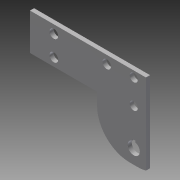
# Autodesk Inventor part: M - arm mount
Saved by Autodesk Inventor 2013 (Build 170138000, 138)
## iProperties
Created: 2013-01-24
Part Number: M - arm mount
Material: Steel
Document SubType Name: Sheet Metal
Designer: Arpan
Density: 7.85 g/cm^3
Sheet Metal Rule: Default
Mass: 87.6442 g
Surface Area: 84.0114 cm^2
Volume: 11.1649 cm^3
Author: Arpan
Autodesk Inventor part; units mm, degrees
ref_plane "YZ Plane" through (0, 0, 0) normal (1, 0, 0) x (0, 1, 0)
ref_plane "XZ Plane" through (0, 0, 0) normal (0, 1, 0) x (-1, 0, 0)
sketch "Sketch1" plane through (0, 0, 0) normal (0, 0, 1) x (1, 0, 0)
  line L0 (-56.9976, 63.5) -> (0, 63.5)
  line L1 (0, 63.5) -> (-7.493, 63.5)
  line L2 (-7.493, 63.5) -> (-7.493, 57.15)
  line L3 (-56.9976, 63.5) -> (-49.5046, 63.5)
  line L4 (-49.5046, 63.5) -> (-49.5046, 57.15)
  line L5 (-56.9976, 63.5) -> (-56.9976, 0)
  line L6 (-56.9976, 0) -> (0, 0)
  line L7 (0, 0) -> (0, 63.5)
  line L8 (-28.4988, 0) -> (-28.4988, 11.1125)
  circle A0 centre (-28.4988, 11.1125) radius 4.7625
  dimension "d3" = 7.493
  dimension "d4" = 6.35
  dimension "d5" = 7.493
  dimension "d19" = 6.35
  dimension "d60" = 63.5
  dimension "d61" = 11.1125
  dimension "d62" = 9.525
  constraints: 18 end point, 3 perpendicular, 2 point on line, 1 centre point, 1 coincident, 1 midpoint, 1 parallel
  measures "d3" distance of L0.end L1.end
  measures "d4" distance of L1.end L2.end
  measures "d5" distance of L0.start L3.end
  measures "d19" distance of L3.end L4.end
  measures "d60" distance of L0.start L5.end
  measures "d61" distance of L8.start L8.end
  measures "d62" diameter of A0
extrude "Plate6" add sketch "Sketch1" along normal blind 3.175
sketch "Sketch6" plane through (0, 0, 0) normal (0, 0, -1) x (-1, 0, 0)
  line L0 (56.9976, 63.5) -> (56.9976, 0) projected
  line L1 (28.4988, 11.1125) -> (27.3076, 11.1125)
  line L2 (28.4988, 11.1125) -> (29.6894, 11.1125)
  circle A0 centre (28.4988, 11.1125) radius 4.7625
  circle A1 centre (28.4988, 11.1125) radius 4.7625 projected
  line L3 (27.3076, 11.1125) -> (29.6888, 11.1125)
  line L4 (29.6888, 11.1125) -> (29.6888, 15.7239)
  line L5 (29.6888, 15.7239) -> (27.3076, 15.7239)
  line L6 (27.3076, 15.7239) -> (27.3076, 11.1125)
  line L7 (27.3076, 15.7239) -> (27.3076, 16.9145)
  line L8 (27.3076, 16.9145) -> (29.6888, 16.9145)
  line L9 (29.6888, 16.9145) -> (29.6888, 15.7239)
  point P0 (27.2012, 15.6948)
  point P1 (30.5454, 15.4129)
  dimension "d82" = 1.1906
  dimension "d86" = 2.3813
  dimension "d87" = 1.1906
  constraints: 18 end point, 6 point on circle, 4 perpendicular, 2 collinear, 2 parallel, 1 centre point, 1 coincident, 1 horizontal
  measures "d82" distance of L1.start L2.end
  measures "d86" distance between parallel lines of L4 L6
  measures "d87" distance of L5.end L7.end
extrude "Cut1" cut sketch "Sketch6" against normal blind 3.175 contours L7 L8 L9 A0 | A0 L5
sketch "Sketch7" plane through (-56.9976, 0, 0) normal (-1, 0, 0) x (0, 0, 1)
  line L0 (3.175, 0) -> (3.175, 63.5) projected
  line L1 (0, 63.5) -> (3.175, 63.5) projected
  line L2 (0, 63.5) -> (0, 0) projected
  line L3 (0, 0) -> (3.175, 0) projected
extrude "Extrusion2" add sketch "Sketch7" along normal blind 52.1462
sketch "Sketch8" plane through (0, 0, 3.175) normal (0, 0, 1) x (1, 0, 0)
  line L0 (0, 0) -> (-109.1438, 0) projected
  line L1 (-109.1438, 0) -> (-109.1438, 63.5) projected
  line L2 (-109.1438, 63.5) -> (-109.1438, 34.925)
  line L3 (-109.1438, 34.925) -> (-56.9976, 34.925)
  line L4 (-56.9976, 34.925) -> (-56.9976, 0)
  circle A0 centre (-75.5412, 57.15) radius 3.3782 projected
  circle A1 centre (-75.5412, 41.275) radius 3.3782 projected
  dimension "d71" = 28.575
  dimension "d72" = 52.1462
  constraints: 6 end point, 2 perpendicular, 2 point on line
  measures "d71" distance of L1.end L2.end
  measures "d72" distance of L2.end L3.end
sketch "Sketch9" plane through (0, 0, 0) normal (0, 0, -1) x (-1, 0, 0)
  circle A0 centre (49.4976, 57.2287) radius 3.3
  circle A1 centre (7.4976, 57.2287) radius 3.3
  constraints: 2 centre point, 4 other
extrude "Cut3" cut sketch "Sketch9" against normal blind 3.175
extrude "Cut4" cut sketch "Sketch8" against normal blind 3.175 contours L0 L1 L3 L4
sketch "Sketch10" plane through (0, 0, 3.175) normal (0, 0, 1) x (1, 0, 0)
  circle A0 centre (-90.6002, 57.15) radius 3.3782 projected
  circle A1 centre (-90.6002, 41.275) radius 3.3782 projected
extrude "Cut5" cut sketch "Sketch10" against normal blind 3.175
fillet "Fillet1" radius 25.4 2 edges at (-56.9976, 0, 1.5875) (0, 0, 1.5875)
sketch "Sketch11" plane through (0, 0, 3.175) normal (0, 0, 1) x (1, 0, 0)
  circle A0 centre (-90.6002, 57.15) radius 3.3782 projected
  circle A1 centre (-90.6002, 41.275) radius 3.3782 projected
  arc A2 (-25.4, 0) -> (0, 25.4) centre (-25.4, 25.4) ccw projected
  line L0 (0, 63.5) -> (0, 25.4) projected
  line L1 (-109.1438, 63.5) -> (0, 63.5) projected
  line L2 (-109.1438, 34.925) -> (-109.1438, 63.5) projected
  line L3 (-109.1438, 34.925) -> (-56.9976, 34.925) projected
  line L4 (-56.9976, 34.925) -> (-56.9976, 25.4) projected
  arc A3 (-56.9976, 25.4) -> (-31.5976, 0) centre (-31.5976, 25.4) ccw projected
  line L5 (-25.4, 0) -> (-31.5976, 0) projected
  circle A4 centre (-49.4976, 57.2287) radius 3.3 projected
  circle A5 centre (-7.4976, 57.2287) radius 3.3 projected
  line L6 (-29.6888, 15.7239) -> (-29.6888, 16.9145) projected
  line L7 (-29.6888, 16.9145) -> (-27.3076, 16.9145) projected
  line L8 (-27.3076, 16.9145) -> (-27.3076, 15.7239) projected
  line L9 (-27.3076, 15.7239) -> (-27.3088, 15.7239) projected
  arc A6 (-29.6888, 15.7239) -> (-27.3088, 15.7239) centre (-28.4988, 11.1125) ccw projected
  point P0 (0, 0)
ref_plane "Work Plane2" through (-28.4982, 16.9145, 3.175) normal (1, 0, 0) x (0, 0, -1)
sketch "Sketch12" plane through (0, 0, 0) normal (0, 0, -1) x (-1, 0, 0)
  arc A0 (0, 25.4) -> (25.4, 0) centre (25.4, 25.4) ccw projected
  line L0 (0, 63.5) -> (109.1438, 63.5) projected
  line L1 (0, 25.4) -> (0, 63.5) projected
  line L2 (27.3076, 16.9145) -> (29.6888, 16.9145) projected
  circle A1 centre (7.4976, 57.2287) radius 3.3 projected
  circle A2 centre (28.4982, 58.7375) radius 3.175 projected
  circle A3 centre (28.4982, 39.6875) radius 3.175 projected
  line L3 (19.05, 63.5) -> (19.05, 0.8066)
  point P0 (0, 0)
  dimension "d88" = 19.05
  constraints: 2 end point, 1 perpendicular, 1 point on circle, 1 point on line
  measures "d88" distance between parallel lines of L3 L1
extrude "Cut6" cut sketch "Sketch12" against normal blind 3.175
equation "\"d67\" = Thickness"
equation "\"d75\" = Thickness"
equation "\"d77\" = Thickness"
equation "\"d79\" = Thickness"
equation "\"d89\" = Thickness"
equation "\"BendRadius\" = Thickness"
equation "\"BendReliefWidth\" = Thickness"
equation "\"BendReliefDepth\" = 0.5 * Thickness"
equation "\"CornerReliefSize\" = 4 * Thickness"
equation "\"MinimumRemnant\" = 2 * Thickness"
equation "\"TransitionRadius\" = BendRadius"
equation "\"JacobiRadiusSize\" = BendRadius"
equation "\"GapSize\" = Thickness"
equation "\"d8\" = BendRadius"
equation "\"d56\" = BendRadius"
equation "\"d63\" = BendRadius"
equation "\"Thickness\" = 3.175"
body "Solid3"
